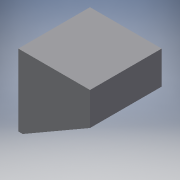
# Autodesk Inventor part: Tool_Mount
Saved by Autodesk Inventor 2019 (Build 230136000, 136)
## iProperties
Created: 2021-01-18
Part Number: Tool_Mount
Material: Generic
Document SubType Name: Modeling
Designer: zhanb
Density: 1 g/cm^3
Appearance: Default
Author: zhanb
Autodesk Inventor part; units mm, degrees
ref_plane "YZ Plane" through (0, 0, 0) normal (1, 0, 0) x (0, 1, 0)
ref_plane "XZ Plane" through (0, 0, 0) normal (0, 1, 0) x (-1, 0, 0)
ref_plane "XY Plane" through (0, 0, 0) normal (0, 0, 1) x (1, 0, 0)
sketch "Sketch2" plane through (0, 0, 0) normal (0, 0, 1) x (1, 0, 0)
  line L0 (-25.4, 25.4) -> (25.4, 25.4)
  line L1 (25.4, 25.4) -> (25.4, 2.0963)
  line L2 (25.4, -25.4) -> (-22.225, -25.4) construction
  line L3 (-25.4, -25.4) -> (-25.4, 25.4)
  line L4 (-25.4, 25.4) -> (25.4, -25.4) construction
  line L5 (25.4, 25.4) -> (-25.4, -25.4) construction
  line L6 (25.4, 2.0963) -> (25.4, -25.4) construction
  line L7 (25.4, 2.0963) -> (-22.225, -25.4)
  line L8 (-22.225, -25.4) -> (-25.4, -25.4)
  point P0 (0, 0)
  dimension "d5" = 30
  dimension "d6" = 3.175
  dimension "d7" = 50.8
  dimension "d8" = 50.8
  constraints: 18 end point, 4 parallel, 2 midpoint, 2 perpendicular, 1 horizontal
  measures "d5" angle of L2 L7
  measures "d6" distance of L2.end L3.start
  measures "d7" distance of L0.start L0.end
  measures "d8" distance of L3.start L0.start
extrude "Extrusion2" add sketch "Sketch2" along normal blind 50.8
sketch "Sketch3" plane through (25.4, 2.0963, 0) normal (0.5, -0.866, 0) x (0.866, 0.5, 0)
  line L0 (0, 0) -> (-54.9926, 0) construction
  line L1 (0, 0) -> (0, 50.8) construction
  line L2 (-54.9926, 50.8) -> (0, 50.8) construction
  line L3 (-54.9926, 0) -> (-54.9926, 50.8) construction
  circle A0 centre (-28.575, 25.4) radius 19.05
  line L4 (0, 0) -> (0, 50.8) construction
  line L5 (0, 25.4) -> (-54.9926, 25.4) construction
  point P0 (-23.0452, 0)
  dimension "d11" = 38.1
  dimension "d12" = 28.575
  constraints: 2 end point, 2 midpoint, 1 centre point, 1 point on line
  measures "d11" diameter of A0
  measures "d12" distance from line of L1 A0.centre
extrude "Extrusion3" cut sketch "Sketch3" against normal blind 12.7
body "Solid2"
